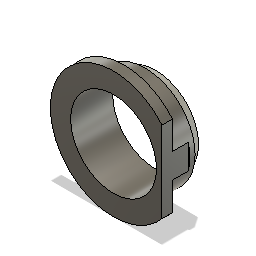
5stack_LED_spacer_8-9.5 (Autodesk Fusion 360 design; units mm, degrees)
Autodesk Fusion 360 part; units mm, degrees
note: some values were not read from the file. Set by a fixed rule: which sketch regions a step uses.
sketch "スケッチ1" plane through (0, 0, 0) normal (0, 1, 0) x (1, 0, 0)
  line L0 (0, 0) -> (-4.07, 0)
  line L1 (-4.07, 0) -> (-4.07, 1)
  line L2 (-4.07, 1) -> (0, 1)
  line L3 (0, 1) -> (0, 0)
  line L4 (-4.07, 1) -> (-6, 1)
  line L5 (-6, 1) -> (-6, 0)
  line L6 (-6, 0) -> (-4.07, 0)
  line L7 (-4.07, 0) -> (-4.07, 1)
  line L8 (-4.07, 1) -> (-4.07, 3)
  line L9 (-4.07, 3) -> (-4.75, 1)
  line L10 (-4.75, 1) -> (-4.07, 1)
  line L11 (-4.07, 1) -> (-4.07, 3)
  line L12 (-4.07, 3) -> (-4.75, 3)
  line L13 (-4.75, 3) -> (-4.75, 1)
  line L14 (-4.75, 3) -> (-4.07, 4)
  line L15 (-4.07, 4) -> (-4.07, 3)
  dimension "d2" = 1
  dimension "d3" = 4.07
  dimension "d5" = 6
  dimension "d6" = 2
  dimension "d12" = 1
  dimension "d13" = 0.68
  dimension "d14" = 1.4
  dimension "d15" = 4.75
  constraint horizontal L0
  constraint vertical L1
  constraint horizontal L2
  constraint vertical L3
  constraint coincident L0.start L3.end
  constraint horizontal L4
  constraint vertical L5
  constraint horizontal L6
  constraint vertical L7
  constraint collinear L0 L6
  constraint perpendicular L2 L8
  constraint horizontal L10
  constraint vertical L11
  constraint horizontal L12
  constraint vertical L13
  constraint collinear L8 L15
  constraint collinear L4 L10
  measures "d2" distance of L0.start L2.end
  measures "d3" distance of L0.start L0.end
  measures "d5" distance of L0.start L5.end
  measures "d6" distance of L1.end L8.end
  measures "d12" distance of L8.end L14.end
  measures "d13" distance of L11 L13
  measures "d15" distance of L3 L13
revolve "回転1" add sketch "スケッチ1" angle 360 about axis through (0, 0, -1) along (0, 0, 1) contours L1 L4 L5 L6 L7 L10 | L4 L8 L9 L10 L11 | L9 L12 L13 | L12 L14 L15
sketch "スケッチ2" plane through (0, 0, 0) normal (0, 0, 1) x (1, 0, 0)
  line L0 (6, 6) -> (4.6, 6)
  line L1 (4.6, 6) -> (4.6, -6)
  line L2 (4.6, -6) -> (6, -6)
  line L3 (6, -6) -> (6, 6)
  circle A0 centre (0, 0) radius 6
  dimension "d11" = 1.4
  constraint horizontal L0
  constraint vertical L1
  constraint horizontal L2
  constraint vertical L3
  constraint tangent L3 A0
  constraint tangent L0 A0
  constraint tangent L2 A0
  measures "d11" distance of L0.start L0.end
extrude "押し出し1" cut sketch "スケッチ2" against normal blind 2.5 contours L1 A0 picked at (4.7636, 1.0585)
